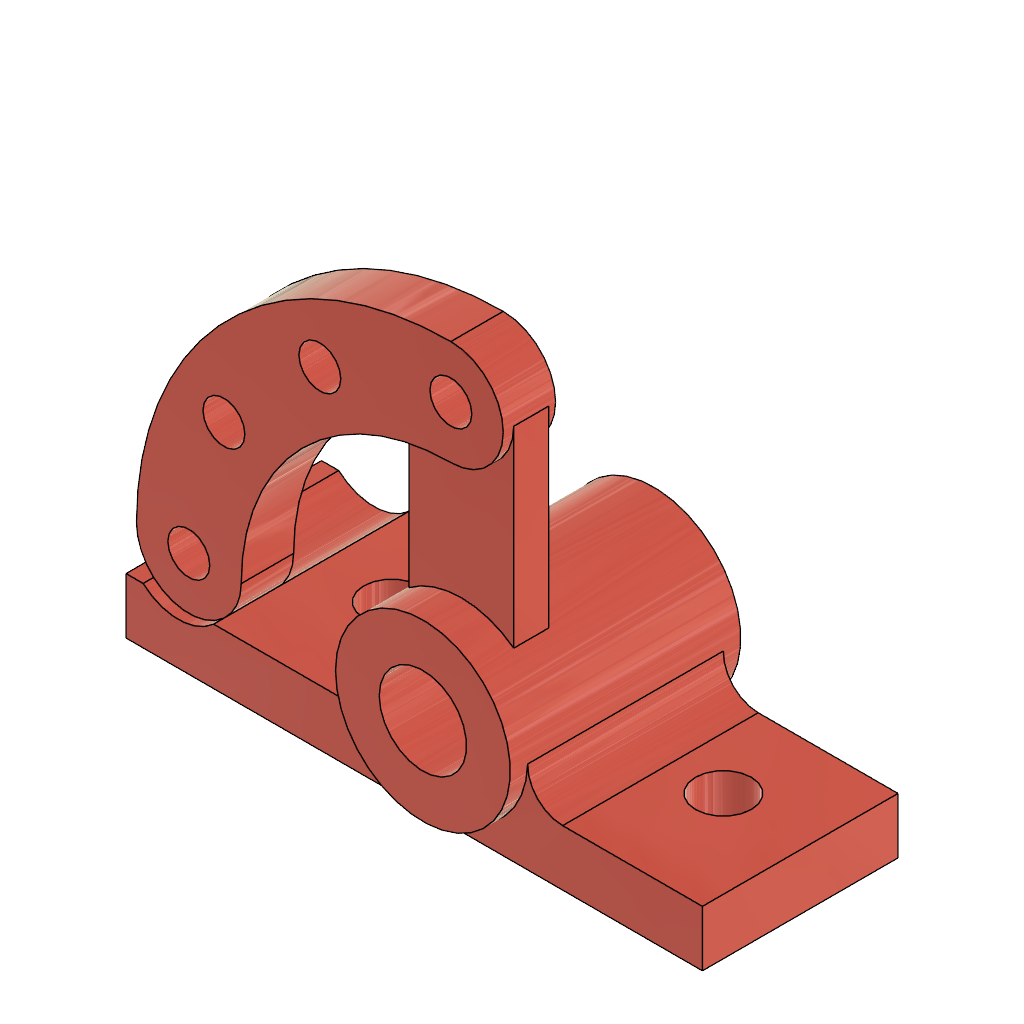
3rd flanged bearing housing (Autodesk Fusion 360 design; units mm, degrees)
part number: 2026-01-11-19-47-32-708
Autodesk Fusion 360 part; units mm, degrees
sketch "Sketch1" plane through (0, 0, 0) normal (0, 1, 0) x (1, 0, 0)
  line L0 (82.5, 8) -> (-82.5, 8)
  line L1 (-82.5, 8) -> (-82.5, -8)
  line L2 (-82.5, -8) -> (82.5, -8)
  line L3 (82.5, -8) -> (82.5, 8)
  line L4 (82.5, 8) -> (-82.5, -8) construction
  line L5 (-82.5, 8) -> (82.5, -8) construction
  circle A0 centre (7.5, -19) radius 12.5
  circle A1 centre (7.5, -19) radius 25
  arc A2 (-52.5, -19) -> (7.5, -79) centre (7.5, -19) ccw
  arc A3 (-82.4998, -19.2063) -> (7.5, -109) centre (7.5, -19) ccw
  circle A4 centre (7.5, -94) radius 15
  circle A5 centre (-67.4999, -19.1031) radius 15.0002
  circle A6 centre (7.5, -94) radius 6
  circle A7 centre (-30, -83.9519) radius 6
  circle A8 centre (-57.4519, -56.5) radius 6
  circle A9 centre (-67.5, -19) radius 6
  line L6 (22.5, -94) -> (22.5, -39)
  line L7 (-7.5, -94) -> (-7.5, -39)
  dimension "d1" = 165
  dimension "d2" = 16
  dimension "d3" = 25
  dimension "d4" = 50
  dimension "d5" = 27
  dimension "d6" = 7.5
  dimension "d7" = 60
  dimension "d8" = 90
  dimension "d9" = 12
  dimension "d11" = -90
  constraint horizontal L0
  constraint perpendicular L0 L1
  constraint parallel L0 L2
  constraint parallel L1 L3
  constraint coincident L4 origin
  constraint coincident L5 origin
  constraint concentric A0 A1
  constraint coincident A0.centre A1.centre
  constraint coincident A3.end A4
  constraint tangent A3 A4
  constraint coincident A2.end A4
  constraint coincident A3.start A5
  constraint coincident A2.start A5
  constraint concentric A4 A6
  constraint coincident A4 L6.start
  constraint tangent A4 L6
  constraint coincident A1 L6.end
  constraint vertical L6
  constraint coincident A4 L7.start
  constraint coincident A1 L7.end
  constraint tangent A4 L7
  constraint parallel L6 L7
  measures "d1" distance of L1.end L2.end
  measures "d2" distance of L0.end L1.end
  measures "d3" diameter of A0
  measures "d4" diameter of A1
  measures "d5" distance of L0 A0.centre
  measures "d6" horizontal distance of origin A0.centre
  measures "d7" radius of A2
  measures "d8" radius of A3
  measures "d9" diameter of A6
extrude "Extrude1" add sketch "Sketch1" along normal mid plane 56 contours L0 L1 L2 L3 A1 A5
extrude "Extrude2" add sketch "Sketch1" along normal mid plane 66 contours L2 A0 A1 | L2 A0 A1
extrude "Extrude3" add sketch "Sketch1" against normal blind 15 from surface at -10 contours L2 A5 | L2 A2 A5 | A2 A3 A4 A5 L7 | A4 | A2 A4 L7
extrude "Extrude4" add sketch "Sketch1" against normal blind 10 from surface at -12 contours A1 A2 A4 L6 L7
hole "Hole1" at (57.5, 3, 8) direction (0, 0, -1) diameter 16 end through all
hole "Hole2" at (-37.4139, 3, 8) direction (0, 0, -1) diameter 16 end through all
fillet "Fillet1" radius 10 1 edges at (29.9499, 0, 8)
